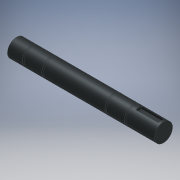
# Autodesk Inventor part: 10PI축
Saved by Autodesk Inventor 2017 (Build 210142000, 142)
## iProperties
Part Number: 10PI축
Material: 철, 주조
Document SubType Name: Modeling
Designer: minom
Density: 7.15 g/cm^3
Appearance: 철 회색
Mass: 43.5695 g
Surface Area: 27.0733 cm^2
Volume: 6.09363 cm^3
Author: minom
Autodesk Inventor part; units mm, degrees
ref_plane "YZ Plane" through (0, 0, 0) normal (1, 0, 0) x (0, 1, 0)
ref_plane "XZ Plane" through (0, 0, 0) normal (0, 1, 0) x (-1, 0, 0)
sketch "스케치1" plane through (0, 0, 0) normal (1, 0, 0) x (0, 1, 0)
  circle A0 centre (0, 0) radius 6
  dimension "d0" = 12
  constraints: 1 centre point, 1 coincident
  measures "d0" diameter of A0
extrude "돌출1" add sketch "스케치1" along normal blind 80
sketch "스케치8" plane through (0, 0, 0) normal (-1, 0, 0) x (0, 0, 1)
  circle A0 centre (0, 0) radius 6 projected
  circle A1 centre (0, 0) radius 4.95
  dimension "d26" = 9.9
  constraints: 1 centre point, 1 coincident
  measures "d26" diameter of A1
extrude "돌출8" cut sketch "스케치8" against normal blind 18.6
sketch "스케치9" plane through (0, 0, 0) normal (-1, 0, 0) x (0, 0, 1)
  circle A0 centre (0, 0) radius 4.8
  circle A1 centre (0, 0) radius 4.95 projected
  dimension "d29" = 9.6
  constraints: 1 centre point, 1 coincident
  measures "d29" diameter of A0
extrude "돌출9" cut sketch "스케치9" against normal blind 9
sketch "스케치10" plane through (0, 0, 0) normal (-1, 0, 0) x (0, 0, 1)
  circle A0 centre (0, 0) radius 4.95
  circle A1 centre (0, 0) radius 4.8 projected
  dimension "d32" = 9.9
  constraints: 1 centre point, 1 coincident
  measures "d32" diameter of A0
extrude "돌출10" add sketch "스케치10" against normal blind 8
sketch "스케치11" plane through (80, 0, 0) normal (1, 0, 0) x (0, 0, -1)
  circle A0 centre (0, 0) radius 6 projected
  circle A1 centre (0, 0) radius 4.95
  dimension "d35" = 9.9
  constraints: 1 centre point, 1 coincident
  measures "d35" diameter of A1
extrude "돌출11" cut sketch "스케치11" against normal blind 26
sketch "스케치12" plane through (80, 0, 0) normal (1, 0, 0) x (0, 0, -1)
  circle A0 centre (0, 0) radius 4.95 projected
  circle A1 centre (0, 0) radius 4.8
  dimension "d38" = 9.6
  constraints: 1 centre point, 1 coincident
  measures "d38" diameter of A1
extrude "돌출12" cut sketch "스케치12" against normal blind 16.4
sketch "스케치13" plane through (80, 0, 0) normal (1, 0, 0) x (0, 0, -1)
  circle A0 centre (0, 0) radius 4.95
  circle A1 centre (0, 0) radius 4.8 projected
  dimension "d41" = 9.9
  constraints: 1 centre point, 1 coincident
  measures "d41" diameter of A0
extrude "돌출13" add sketch "스케치13" against normal blind 15.4
ref_plane "작업 평면1" through (80, 0, 4.95) normal (0, 0, 1) x (1, 0, 0)
sketch "스케치14" plane through (80, 0, 4.95) normal (0, 0, 1) x (1, 0, 0)
  line L0 (-1.3, -1.55) -> (-13.4, -1.55)
  line L1 (-13.4, -1.55) -> (-13.4, 1.55)
  line L2 (-13.4, 1.55) -> (-1.3, 1.55)
  line L3 (-1.3, 1.55) -> (-1.3, -1.55)
  line L4 (-15.4, 4.95) -> (-15.4, -4.95) projected
  line L5 (0, 4.95) -> (0, -4.95) projected
  line L6 (0, 0) -> (-15.4, 0)
  line L7 (-15.4, 4.8) -> (-15.4, -4.8) projected
  point P0 (-80, 0)
  dimension "d44" = 12.1
  dimension "d45" = 3.1
  dimension "d46" = 12.1
  dimension "d47" = 2
  dimension "d48" = 1.55
  constraints: 10 end point, 2 midpoint, 2 perpendicular, 1 horizontal
  measures "d44" distance of L0.start L0.end
  measures "d45" distance of L0.end L1.end
  measures "d46" distance of L1.end L2.end
  measures "d47" distance between parallel lines of L4 L1
  measures "d48" distance between parallel lines of L6 L0
extrude "돌출14" cut sketch "스케치14" against normal blind 1.3
sketch "스케치15" plane through (54, 0, 0) normal (1, 0, 0) x (0, 0, -1)
  circle A0 centre (0, 0) radius 4.95 projected
  circle A1 centre (0, 0) radius 6 projected
  circle A2 centre (0, 0) radius 4.95 projected
  circle A3 centre (0, 0) radius 4.95 projected
  circle A4 centre (0, 0) radius 4.8
  dimension "d51" = 9.6
  constraints: 1 centre point, 1 coincident
  measures "d51" diameter of A4
extrude "돌출15" cut sketch "스케치15" against normal blind 1 contours A0 | A1
sketch "스케치16" plane through (18.6, 0, 0) normal (-1, 0, 0) x (0, 0, 1)
  circle A0 centre (0, 0) radius 4.95 projected
  circle A1 centre (0, 0) radius 6 projected
  circle A2 centre (0, 0) radius 4.95 projected
  circle A3 centre (0, 0) radius 4.8
  dimension "d54" = 9.6
  constraints: 1 centre point, 1 coincident
  measures "d54" diameter of A3
extrude "돌출16" cut sketch "스케치16" against normal blind 1.1 contours A0 | A1
sketch "스케치17" plane through (19.7, 0, 0) normal (-1, 0, 0) x (0, 0, 1)
  circle A0 centre (0, 0) radius 4.8 projected
  circle A1 centre (0, 0) radius 6 projected
  circle A2 centre (0, 0) radius 4.95 projected
  circle A3 centre (0, 0) radius 4.95
  constraints: 1 centre point, 1 coincident
extrude "돌출17" cut sketch "스케치17" against normal blind 33.35 contours A1
